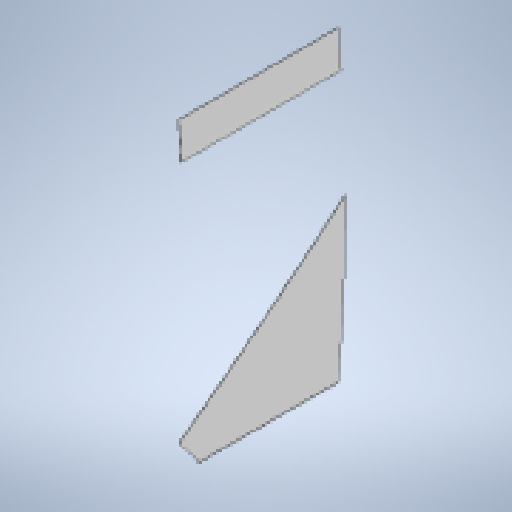
# Autodesk Inventor part: MSC 027 sheet left-right board face 1
Saved by Autodesk Inventor 2025 (Build 290162010, 162A)
## iProperties
Created: 2024-04-18
Part Number: MSC 027 sheet left-right board face 1
Material: AISI304
Document SubType Name: Sheet Metal
Designer: admin
Stock Number: МОО 027 лист левый-правый борт морда 1
Mass: 48027.3 g
Surface Area: 40202.8 cm^2
Volume: 6003.41 cm^3
Density: 8 g/cm^3
Sheet Metal Rule: Default_mm
Sheet Metal Width: 0,000 mm
Sheet Metal Length: 0,000 mm
Sheet Metal Area: 0,000 mm^2
Appearance: Default
Author: admin
Autodesk Inventor part; units mm, degrees
ref_plane "YZ Plane" through (0, 0, 0) normal (1, 0, 0) x (0, 1, 0)
ref_plane "XZ Plane" through (0, 0, 0) normal (0, 1, 0) x (-1, 0, 0)
ref_plane "XY Plane" through (0, 0, 0) normal (0, 0, 1) x (1, 0, 0)
sketch "Sketch1" plane through (0, 0, 0) normal (0, 0, 1) x (1, 0, 0)
  line L0 (394.757121, -1035.809004) -> (394.757121, -1085.809004) construction
  line L1 (0, -1088.809004) -> (0, -1880) construction
  arc A0 (0.159434, -1878.130723) -> (0, 0) centre (-11009.945504, -940) ccw
  arc A1 (0, -1880) -> (0.159434, -1878.130723) centre (-11009.945504, -940) ccw construction
  arc A2 (-1.349222, -1881.302929) -> (0.159434, -1878.130723) centre (-4.822514, -1877.70623) ccw
  line L2 (-1.349222, -1881.302929) -> (0, -1880) construction
  line L3 (-71.93398, -1949.465837) -> (-1.349222, -1881.302929)
  line L4 (-247.746289, -1767.406862) -> (-71.93398, -1949.465837) construction
  line L5 (0, -1880) -> (0, 0) construction
  line L6 (0, -1880) -> (1.875639, -1880) construction
  dimension "d153" = 5
  dimension "d154" = 100
  dimension "d155" = 11050
  dimension "d156" = 136
  dimension "d157" = 1880
  measures "d153" radius of A2
  measures "d154" distance of L1.end L3.start
  measures "d155" radius of A0
  measures "d156" angle of L2 L6
  measures "d157" distance of L1.end L5.end
contour flange "Contour Flange2" sketch "Sketch1" thickness 3 bend radius 3 width 980 along (0, 0, 1) mid plane no both sides no wall seen from (-36.641601, -1915.384383, 0) lies toward (0.6946584, -0.7193398, 0) curves L3 A2 A0
bend "Bend2"
corner "Corner2"
sketch "Sketch2" plane through (0, 0, 0) normal (1, 0, 0) x (0, 1, 0)
  line L0 (-2098.410388, 980) -> (-2098.410388, 0)
  line L1 (-2098.410388, 0) -> (-216.673819, 0)
  line L2 (-216.673819, 0) -> (-216.673819, 980)
  line L3 (-2098.410388, 980) -> (-216.673819, 980)
  line L4 (-2103.474264, 980) -> (-2103.474264, 0)
  line L5 (-2165.821082, 980) -> (-2103.474264, 980)
  line L6 (-2165.821082, 0) -> (-2165.821082, 980)
  line L7 (-2165.821082, 0) -> (-2103.474264, 0)
  line L8 (-2098.410388, 0) -> (-2103.474264, 0)
  line L9 (-2098.410388, 980) -> (-2103.474264, 980)
  line L10 (-871.885819, 980) -> (-1694.203458, 0)
  line L11 (-871.885819, 0) -> (-1694.203458, 980)
  line L12 (-1722.439791, 980) -> (-2165.821082, 607.958923)
  line L13 (-1722.439791, 0) -> (-2165.821082, 372.041077)
  point P0 (0, 0)
  point P1 (-1283.044638, 490)
  dimension "d150" = 40
  dimension "d151" = 285
  dimension "d152" = 655.212
  constraints: 12 end point, 8 point on line, 2 equal length, 2 midpoint, 2 perpendicular, 1 horizontal
  measures "d150" angle of L3 L12
  measures "d151" distance from line of L12 L5.start
  measures "d152" distance of L11.start L1.end
extrude "Extrusion2" cut sketch "Sketch2" along normal through all both and the other way through all contours L3 L12 L0 | L0 L12 L4 L9 | L4 L12 L6 L5 | L3 L10 L11 | L3 L2 L1 L11 L10
sketch "Sketch4" plane through (749.1768, -2100.77463, 662.50511) normal (-0.6852958, 0.7282648, 0) x (0.7282648, 0.6852958, 0)
  line L0 (-59.382943, 165.716241) -> (-59.382943, 507.035792) construction
  line L1 (-59.382943, 507.035792) -> (-32.420537, 507.035792) construction
  line L2 (-32.420537, 507.035792) -> (-32.420537, 165.716241) construction
  line L3 (-32.420537, 165.716241) -> (-59.382943, 165.716241) construction
  point P0 (894.052911, 662.50511)
  constraints: 2 other
feature "Mark2" [suppressed]
equation "\"d36\" = Thickness"
equation "\"d37\" = BendReliefWidth"
equation "\"d38\" = BendReliefDepth"
equation "\"d39\" = MinimumRemnant"
equation "\"d40\" = TransitionRadius"
equation "\"d42\" = BendRadius"
equation "\"d44\" = CornerReliefSize"
equation "\"d45\" = GapSize"
equation "\"d46\" = JacobiRadiusSize"
equation "\"BendRadius\" = Thickness"
equation "\"BendReliefWidth\" = Thickness"
equation "\"BendReliefDepth\" = 0.5 * Thickness"
equation "\"CornerReliefSize\" = 4 * Thickness"
equation "\"MinimumRemnant\" = 2 * Thickness"
equation "\"TransitionRadius\" = BendRadius"
equation "\"JacobiRadiusSize\" = BendRadius"
equation "\"GapSize\" = Thickness"
equation "\"Thickness\" = 3"
body "Solid3"
